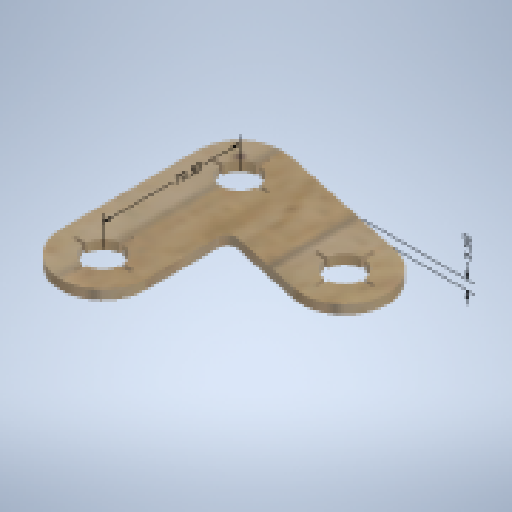
# Autodesk Inventor part: gear_plate_1
Saved by Autodesk Inventor 2024.1 (Build 281209000, 209)
## iProperties
Created: 2024-04-01
Part Number: gear_plate_1
Material: 木材 (カエデ材)
Document SubType Name: Modeling
Designer: hibik
Density: 0.67 g/cm^3
Appearance: ナチュラル カエデ材 - 光沢 濃い着色
Author: hibik
Autodesk Inventor part; units mm, degrees
ref_plane "YZ Plane" through (0, 0, 0) normal (1, 0, 0) x (0, 1, 0)
ref_plane "XZ Plane" through (0, 0, 0) normal (0, 1, 0) x (-1, 0, 0)
ref_plane "XY Plane" through (0, 0, 0) normal (0, 0, 1) x (1, 0, 0)
sketch "スケッチ1" plane through (0, 0, 0) normal (0, 1, 0) x (-1, 0, 0)
  line L0 (25, 0) -> (-25, 0)
  line L1 (-25, 0) -> (-25, -104.5)
  line L2 (-25, -104.5) -> (25, -104.5) construction
  line L3 (25, -104.5) -> (25, 0)
  circle A0 centre (0, 0) radius 25
  circle A1 centre (0, 0) radius 57 construction
  circle A2 centre (0, -79.5) radius 22.5 construction
  circle A3 centre (0, 0) radius 75 construction
  circle A4 centre (0, -79.5) radius 10.75
  circle A5 centre (0, 0) radius 10.75
  circle A6 centre (-77.7461, -62.8931) radius 25
  circle A7 centre (-77.7461, -62.8931) radius 10.75
  circle A8 centre (0, -79.5) radius 25
  line L4 (-5.2223, -103.9485) -> (-82.9684, -87.3415)
  line L5 (-72.5238, -38.4446) -> (5.2223, -55.0515)
  line L6 (-77.7461, -62.8931) -> (-82.9684, -87.3415)
  point P0 (25, -79.5)
  point P1 (-25, -48.5959)
  dimension "d0" = 114
  dimension "d1" = 45
  dimension "d2" = 150
  dimension "d4" = 21.5
  dimension "d5" = 50
  dimension "d25" = 79.5
  constraints: 14 end point, 9 centre point, 9 tangent, 8 coincident, 5 point on circle, 3 equal radius, 2 parallel, 2 perpendicular, 1 horizontal, 1 midpoint, 1 vertical alignment
  measures "d0" diameter of A1
  measures "d1" diameter of A2
  measures "d2" diameter of A3
  measures "d4" diameter of A5
  measures "d5" distance of L1.end L2.end
  measures "d25" distance from line of A2.centre L6
extrude "押し出し1" add sketch "スケッチ1" along normal blind 5.5 contours A0 L0 A5 | L0 A5 A0 | L3 A8 L5 L1 A0 | A8 | A8 L1 L5 | L4 L1 A8 | L1 L4 A6 L5 | A6
sketch "スケッチ4" plane through (0, 5.5, 0) normal (0, 1, 0) x (1, 0, 0)
  line L0 (-1, 90.2034) -> (1, 90.2034)
  line L1 (1, 90.2034) -> (1, 96.5)
  line L2 (1, 96.5) -> (-1, 96.5)
  line L3 (-1, 96.5) -> (-1, 90.2034)
  arc A0 (-25, 0) -> (25, 0) centre (0, 0) ccw projected
  line L4 (25, 0) -> (25, 48.5959) projected
  line L5 (25, 48.5959) -> (72.5238, 38.4446) projected
  arc A1 (72.5238, 38.4446) -> (82.9684, 87.3415) centre (77.7461, 62.8931) ccw projected
  line L6 (82.9684, 87.3415) -> (5.2223, 103.9485) projected
  arc A2 (5.2223, 103.9485) -> (-25, 79.5) centre (0, 79.5) ccw projected
  line L7 (-25, 79.5) -> (-25, 0) projected
  circle A3 centre (0, 0) radius 10.75 projected
  circle A4 centre (77.7461, 62.8931) radius 10.75 projected
  circle A5 centre (0, 79.5) radius 10.75 projected
  circle A6 centre (0, 79.5) radius 10.75 projected
  line L8 (-16.9706, -1) -> (16.9706, -1)
  line L9 (16.9706, -1) -> (16.9706, 1)
  line L10 (16.9706, 1) -> (-16.9706, 1)
  line L11 (-16.9706, 1) -> (-16.9706, -1)
  line L12 (-1, -16.9706) -> (1, -16.9706)
  line L13 (1, -16.9706) -> (1, 16.9706)
  line L14 (1, 16.9706) -> (-1, 16.9706)
  line L15 (-1, 16.9706) -> (-1, -16.9706)
  circle A7 centre (0, 0) radius 17
  line L16 (94.7167, 63.8931) -> (60.7756, 63.8931)
  line L17 (60.7756, 63.8931) -> (60.7756, 61.8931)
  line L18 (60.7756, 61.8931) -> (94.7167, 61.8931)
  line L19 (94.7167, 61.8931) -> (94.7167, 63.8931)
  line L20 (78.7461, 79.8636) -> (76.7461, 79.8636)
  line L21 (76.7461, 79.8636) -> (76.7461, 45.9225)
  line L22 (76.7461, 45.9225) -> (78.7461, 45.9225)
  line L23 (78.7461, 45.9225) -> (78.7461, 79.8636)
  line L24 (16.9706, 80.5) -> (-16.9706, 80.5)
  line L25 (-16.9706, 80.5) -> (-16.9706, 78.5)
  line L26 (-16.9706, 78.5) -> (16.9706, 78.5)
  line L27 (16.9706, 78.5) -> (16.9706, 80.5)
  line L28 (16.9706, 80.5) -> (-16.9706, 78.5) construction
  line L29 (-16.9706, 80.5) -> (16.9706, 78.5) construction
  point P0 (0, 96.5)
  point P1 (-16.9706, 0)
  point P2 (0, 16.9706)
  point P3 (-1, -10.7034)
  point P4 (1, -10.7034)
  point P5 (10.7034, 1)
  point P6 (10.7034, -1)
  point P7 (-1, 10.7034)
  point P8 (1, 10.7034)
  point P9 (-10.7034, -1)
  point P10 (-10.7034, 1)
  point P11 (60.7756, 62.8931)
  point P12 (77.7461, 45.9225)
  point P13 (77.7461, 61.8931)
  point P14 (76.7461, 62.8931)
  point P15 (88.4495, 63.8931)
  point P16 (78.7461, 73.5965)
  point P17 (76.7461, 73.5965)
  point P18 (67.0427, 63.8931)
  point P19 (67.0427, 61.8931)
  point P20 (76.7461, 52.1897)
  point P21 (78.7461, 52.1897)
  point P22 (88.4495, 61.8931)
  dimension "d26" = 17
  dimension "d27" = 2
  dimension "d30" = 34
  constraints: 52 end point, 12 parallel, 9 midpoint, 8 equal length, 6 horizontal, 6 perpendicular, 4 point on circle, 4 vertical alignment, 3 horizontal alignment, 1 centre point, 1 coincident, 2 other
  measures "d26" distance from line of L2 A2.centre
  measures "d27" distance of L1.end L2.end
  measures "d30" diameter of A7
extrude "押し出し4" cut sketch "スケッチ4" against normal through all contours A5 L0 | L3 L2 L1 A5 | L24 A5 L26 | A5 L26 L25 L24 | L24 L27 L26 A5 | A3 L10 L9 L8 | A3 L15 L14 L13 | L13 L12 L15 A3 | A3 L8 L11 L10 | A4 L18 L23 L16 | A4 L16 L19 L18 | L16 L23 A4 | A4 L23 L18 | L23 L16 L21 A4 | A4 L21 L20 L23 | L23 L18 L21 L16 | L23 L22 L21 A4 | A4 L21 L18 L23 | L21 L16 A4 | L21 L18 A4 L16 | A4 L18 L21 | A4 L18 L17 L16
fillet "フィレット1" radius 5 1 edges at (25, 2.75, -48.5959)
